Autodesk Fusion 360 part; units mm, degrees
(part 14 of 25)
  arc A3423 (31.4192, 17.8599) -> (31.5407, 18.1532) centre (31.4799, 18.0065) ccw
  line L1201 (39.8479, 17.8026) -> (39.6555, 17.6628)
  arc A3424 (36.7177, 17.8488) -> (36.9423, 17.6243) centre (36.83, 17.7366) ccw
  arc A3425 (41.043, 18.1351) -> (40.9448, 17.8331) centre (40.9939, 17.9841) ccw
  line L1202 (37.7489, 18.2753) -> (37.1, 18.0065)
  line L1203 (38.4511, 18.2753) -> (37.7489, 18.2753)
  arc A3426 (39.7677, 17.5505) -> (39.5432, 17.775) centre (39.6555, 17.6627) ccw
  arc A3427 (40.64, 18.18) -> (40.64, 17.8625) centre (40.64, 18.0212) ccw
  arc A3428 (40.7988, 18.0213) -> (40.4813, 18.0213) centre (40.6401, 18.0213) ccw
  arc A3429 (38.5119, 18.422) -> (38.3904, 18.1286) centre (38.4511, 18.2753) ccw
  arc A3430 (40.64, 16.3513) -> (40.64, 16.6688) centre (40.64, 16.51) ccw
  arc A3431 (40.5459, 17.8645) -> (40.4962, 18.1781) centre (40.5211, 18.0213) ccw
  arc A3432 (40.2613, 18.1409) -> (40.3109, 17.8273) centre (40.2861, 17.9841) ccw
  line L1204 (40.9939, 17.9841) -> (40.7589, 18.0213)
  arc A3433 (41.9212, 17.5879) -> (41.6643, 17.4012) centre (41.7927, 17.4945) ccw
  arc A3434 (40.9691, 17.8273) -> (41.0187, 18.1409) centre (40.9939, 17.9841) ccw
  line L1205 (35.9111, 18.2753) -> (35.2089, 18.2753)
  arc A3435 (27.5889, 18.434) -> (27.5889, 18.1165) centre (27.5889, 18.2752) ccw
  arc A3436 (26.5577, 17.6243) -> (26.7823, 17.8488) centre (26.67, 17.7366) ccw
  arc A3437 (29.0522, 18.1188) -> (28.8277, 17.8943) centre (28.94, 18.0065) ccw
  arc A3438 (30.8311, 18.1165) -> (30.8311, 18.434) centre (30.8311, 18.2752) ccw
  arc A3439 (36.7177, 17.6243) -> (36.9423, 17.8488) centre (36.83, 17.7366) ccw
  arc A3440 (36.6722, 18.1188) -> (36.4477, 17.8943) centre (36.56, 18.0066) ccw
  arc A3441 (29.0977, 17.8488) -> (29.3223, 17.6243) centre (29.21, 17.7366) ccw
  arc A3442 (28.3519, 18.422) -> (28.2304, 18.1286) centre (28.2911, 18.2753) ccw
  arc A3443 (33.9592, 17.8599) -> (34.0807, 18.1532) centre (34.02, 18.0065) ccw
  arc A3444 (33.4319, 18.422) -> (33.3104, 18.1286) centre (33.3712, 18.2753) ccw
  line L1206 (31.48, 18.0065) -> (30.8311, 18.2753)
  line L1207 (26.67, 17.7365) -> (26.4, 18.0065)
  line L1208 (28.94, 18.0065) -> (28.2911, 18.2753)
  line L1209 (32.6689, 18.2753) -> (32.02, 18.0065)
  arc A3445 (32.1323, 17.8943) -> (31.9078, 18.1188) centre (32.0201, 18.0066) ccw
  line L1210 (28.2911, 18.2753) -> (27.5889, 18.2753)
  arc A3446 (31.9593, 18.1532) -> (32.0808, 17.8599) centre (32.0201, 18.0066) ccw
  arc A3447 (34.1322, 18.1188) -> (33.9077, 17.8943) centre (34.02, 18.0066) ccw
  arc A3448 (35.2089, 18.434) -> (35.2089, 18.1165) centre (35.2089, 18.2752) ccw
  arc A3449 (26.8793, 18.1532) -> (27.0008, 17.8599) centre (26.9401, 18.0065) ccw
  line L1211 (34.29, 17.7365) -> (34.02, 18.0065)
  arc A3450 (32.7296, 18.1286) -> (32.6081, 18.422) centre (32.6688, 18.2753) ccw
  arc A3451 (30.1896, 18.1286) -> (30.0681, 18.422) centre (30.1288, 18.2753) ccw
  arc A3452 (30.8919, 18.422) -> (30.7704, 18.1286) centre (30.8312, 18.2753) ccw
  line L1212 (34.56, 18.0065) -> (34.29, 17.7365)
  arc A3453 (29.5923, 17.8943) -> (29.3678, 18.1188) centre (29.4801, 18.0066) ccw
  line L1213 (30.1289, 18.2753) -> (29.48, 18.0065)
  line L1214 (29.48, 18.0065) -> (29.21, 17.7365)
  line L1215 (36.83, 17.7365) -> (36.56, 18.0065)
  arc A3454 (35.9111, 18.1165) -> (35.9111, 18.434) centre (35.9111, 18.2752) ccw
  arc A3455 (35.9719, 18.422) -> (35.8504, 18.1286) centre (35.9112, 18.2753) ccw
  arc A3456 (33.3711, 18.1165) -> (33.3711, 18.434) centre (33.3711, 18.2752) ccw
  line L1216 (35.2089, 18.2753) -> (34.56, 18.0065)
  arc A3457 (26.5122, 18.1188) -> (26.2877, 17.8943) centre (26.4, 18.0066) ccw
  arc A3458 (34.1777, 17.6243) -> (34.4023, 17.8488) centre (34.29, 17.7366) ccw
  line L1217 (34.02, 18.0065) -> (33.3711, 18.2753)
  arc A3459 (16.3815, 13.6963) -> (16.26, 13.9897) centre (16.3208, 13.843) ccw
  arc A3460 (31.6377, 17.8488) -> (31.8623, 17.6243) centre (31.75, 17.7366) ccw
  line L1218 (15.9006, 13.669) -> (15.5791, 13.3475)
  line L1219 (27.5889, 18.2753) -> (26.94, 18.0065)
  arc A3461 (15.4669, 13.4597) -> (15.6914, 13.2352) centre (15.5792, 13.3475) ccw
  arc A3462 (28.2911, 18.1165) -> (28.2911, 18.434) centre (28.2911, 18.2752) ccw
  line L1220 (21.3635, 15.51) -> (21.717, 15.1565)
  line L1221 (36.56, 18.0065) -> (35.9111, 18.2753)
  arc A3463 (28.8792, 17.8599) -> (29.0007, 18.1532) centre (28.94, 18.0065) ccw
  line L1222 (32.02, 18.0065) -> (31.75, 17.7365)
  line L1223 (26.4, 18.0065) -> (25.7511, 18.2753)
  arc A3464 (31.6377, 17.6243) -> (31.8623, 17.8488) centre (31.75, 17.7366) ccw
  arc A3465 (29.4193, 18.1532) -> (29.5408, 17.8599) centre (29.4801, 18.0065) ccw
  line L1224 (30.8311, 18.2753) -> (30.1289, 18.2753)
  arc A3466 (36.4992, 17.8599) -> (36.6207, 18.1532) centre (36.56, 18.0065) ccw
  arc A3467 (35.2696, 18.1286) -> (35.1481, 18.422) centre (35.2088, 18.2753) ccw
  arc A3468 (27.0523, 17.8943) -> (26.8278, 18.1188) centre (26.9401, 18.0066) ccw
  arc A3469 (29.0977, 17.6243) -> (29.3223, 17.8488) centre (29.21, 17.7366) ccw
  arc A3470 (30.1289, 18.434) -> (30.1289, 18.1165) centre (30.1289, 18.2752) ccw
  arc A3471 (31.5922, 18.1188) -> (31.3677, 17.8943) centre (31.4799, 18.0066) ccw
  line L1225 (33.3711, 18.2753) -> (32.6689, 18.2753)
  arc A3472 (34.4993, 18.1532) -> (34.6208, 17.8599) centre (34.5601, 18.0065) ccw
  arc A3473 (25.7511, 18.1165) -> (25.7511, 18.434) centre (25.7511, 18.2752) ccw
  arc A3474 (23.9722, 18.1188) -> (23.7477, 17.8943) centre (23.86, 18.0065) ccw
  line L1226 (25.0489, 18.2753) -> (24.4, 18.0065)
  arc A3475 (16.0129, 13.5567) -> (15.7884, 13.7812) centre (15.9007, 13.6689) ccw
  line L1227 (21.0947, 16.8611) -> (21.0947, 16.1589)
  arc A3476 (21.9723, 17.8943) -> (21.7478, 18.1188) centre (21.8601, 18.0066) ccw
  arc A3477 (21.7993, 18.1532) -> (21.9208, 17.8599) centre (21.8601, 18.0065) ccw
  arc A3478 (23.2111, 18.1165) -> (23.2111, 18.434) centre (23.2111, 18.2752) ccw
  line L1228 (14.6499, 12.9032) -> (13.7795, 12.0328)
  arc A3479 (25.8119, 18.422) -> (25.6904, 18.1286) centre (25.7512, 18.2753) ccw
  line L1229 (21.0947, 16.1589) -> (21.3635, 15.51)
  arc A3480 (21.2535, 16.8611) -> (20.9359, 16.8611) centre (21.0947, 16.8611) ccw
  arc A3481 (15.6914, 13.2352) -> (15.4669, 13.4597) centre (15.5792, 13.3475) ccw
  arc A3482 (21.5101, 17.4492) -> (21.2168, 17.5707) centre (21.3635, 17.5099) ccw
  arc A3483 (24.3393, 18.1532) -> (24.4608, 17.8599) centre (24.4001, 18.0065) ccw
  arc A3484 (21.2414, 16.2196) -> (20.948, 16.0981) centre (21.0947, 16.1589) ccw
  line L1230 (23.86, 18.0065) -> (23.2111, 18.2753)
  line L1231 (21.1166, 13.843) -> (16.3207, 13.843)
  arc A3485 (22.5696, 18.1286) -> (22.4481, 18.422) centre (22.5089, 18.2753) ccw
  line L1232 (21.86, 18.0065) -> (21.3635, 17.51)
  arc A3486 (21.8758, 15.1565) -> (21.5583, 15.1565) centre (21.717, 15.1565) ccw
  line L1233 (21.717, 14.4434) -> (21.1166, 13.843)
  arc A3487 (23.2719, 18.422) -> (23.1504, 18.1286) centre (23.2111, 18.2753) ccw
  arc A3488 (22.5089, 18.434) -> (22.5089, 18.1165) centre (22.5089, 18.2752) ccw
  line L1234 (15.5791, 13.3475) -> (15.1349, 12.9032)
  arc A3489 (13.6672, 12.145) -> (13.8918, 11.9205) centre (13.7795, 12.0328) ccw
  arc A3490 (20.948, 16.9219) -> (21.2414, 16.8004) centre (21.0947, 16.8612) ccw
  arc A3491 (13.6208, 10.8018) -> (13.9383, 10.8018) centre (13.7796, 10.8018) ccw
  line L1235 (24.13, 17.7365) -> (23.86, 18.0065)
  line L1236 (21.3635, 17.51) -> (21.0947, 16.8611)
  arc A3492 (21.0043, 13.9553) -> (21.2288, 13.7307) centre (21.1165, 13.843) ccw
  arc A3493 (21.5583, 14.4434) -> (21.8758, 14.4434) centre (21.717, 14.4434) ccw
  arc A3494 (21.8293, 14.3312) -> (21.6047, 14.5557) centre (21.717, 14.4435) ccw
  arc A3495 (21.2168, 15.4493) -> (21.5101, 15.5708) centre (21.3635, 15.51) ccw
  arc A3496 (23.7992, 17.8599) -> (23.9207, 18.1532) centre (23.8599, 18.0065) ccw
  line L1237 (22.5089, 18.2753) -> (21.86, 18.0065)
  arc A3497 (25.0489, 18.434) -> (25.0489, 18.1165) centre (25.0489, 18.2752) ccw
  arc A3498 (24.0177, 17.8488) -> (24.2423, 17.6243) centre (24.13, 17.7366) ccw
  arc A3499 (15.1349, 12.7444) -> (15.1349, 13.0619) centre (15.1349, 12.9032) ccw
  arc A3500 (21.4757, 15.6223) -> (21.2512, 15.3978) centre (21.3635, 15.51) ccw
  arc A3501 (15.8399, 13.8157) -> (15.9614, 13.5223) centre (15.9007, 13.669) ccw
  arc A3502 (14.6499, 13.0619) -> (14.6499, 12.7444) centre (14.6499, 12.9032) ccw
  arc A3503 (24.0177, 17.6243) -> (24.2423, 17.8488) centre (24.13, 17.7366) ccw
  line L1238 (24.4, 18.0065) -> (24.13, 17.7365)
  arc A3504 (20.9359, 16.1589) -> (21.2535, 16.1589) centre (21.0947, 16.1589) ccw
  arc A3505 (26.3392, 17.8599) -> (26.4607, 18.1532) centre (26.3999, 18.0065) ccw
  arc A3506 (15.0226, 13.0155) -> (15.2471, 12.7909) centre (15.1349, 12.9032) ccw
  line L1239 (21.717, 15.1565) -> (21.717, 14.4434)
  line L1240 (25.7511, 18.2753) -> (25.0489, 18.2753)
  arc A3507 (14.7622, 12.7909) -> (14.5377, 13.0155) centre (14.65, 12.9032) ccw
  arc A3508 (25.1096, 18.1286) -> (24.9881, 18.422) centre (25.0489, 18.2753) ccw
  arc A3509 (21.2512, 17.6222) -> (21.4757, 17.3977) centre (21.3635, 17.5099) ccw
  line L1241 (13.7795, 12.0328) -> (13.7795, 10.8018)
  line L1242 (23.2111, 18.2753) -> (22.5089, 18.2753)
  line L1243 (15.1349, 12.9032) -> (14.6499, 12.9032)
  arc A3510 (24.5123, 17.8943) -> (24.2878, 18.1188) centre (24.4001, 18.0066) ccw
  arc A3511 (65.9384, 2.7686) -> (65.9384, 2.7178) centre (65.9384, 2.7432) ccw
  arc A3512 (66.0553, 2.2782) -> (66.0811, 2.2345) centre (66.0682, 2.2564) ccw
  arc A3513 (63.0301, 1.5494) -> (63.0301, 1.6002) centre (63.0301, 1.5748) ccw
  arc A3514 (57.5748, 1.5748) -> (57.6256, 1.5748) centre (57.6002, 1.5748) ccw
  arc A3515 (66.1981, 2.4836) -> (65.9384, 2.7432) centre (65.9384, 2.4835) ccw
  arc A3516 (65.556, 1.8344) -> (65.6068, 1.8344) centre (65.5814, 1.8344) ccw
  arc A3517 (58.2027, 1.5748) -> (58.2535, 1.5748) centre (58.2281, 1.5748) ccw
  line L1244 (55.3077, 1.5748) -> (55.827, 1.5748)
  arc A3518 (55.4375, 2.2493) -> (55.4375, 2.1985) centre (55.4375, 2.2239) ccw
  arc A3519 (65.1543, 2.4836) -> (65.1035, 2.4836) centre (65.1289, 2.4836) ccw
  arc A3520 (58.9026, 2.7432) -> (58.8518, 2.7432) centre (58.8772, 2.7432) ccw
  arc A3521 (55.8524, 2.7432) -> (55.8016, 2.7432) centre (55.827, 2.7432) ccw
  arc A3522 (63.0142, 2.4637) -> (63.046, 2.5034) centre (63.0301, 2.4835) ccw
  line L1245 (54.5067, 2.0941) -> (54.8313, 2.0941)
  arc A3523 (56.6617, 1.5668) -> (56.7099, 1.5828) centre (56.6858, 1.5748) ccw
  arc A3524 (61.238, 1.6002) -> (61.238, 1.5494) centre (61.238, 1.5748) ccw
  line L1246 (57.73, 1.5748) -> (57.4703, 1.5748)
  arc A3525 (55.827, 2.1985) -> (55.827, 2.2493) centre (55.827, 2.2239) ccw
  arc A3526 (54.1594, 1.5862) -> (54.2049, 1.5634) centre (54.1822, 1.5748) ccw
  arc A3527 (55.3077, 1.6002) -> (55.3077, 1.5494) centre (55.3077, 1.5748) ccw
  arc A3528 (54.8313, 2.0687) -> (54.8313, 2.1195) centre (54.8313, 2.0941) ccw
  line L1247 (55.827, 1.5748) -> (55.827, 2.7432)
  arc A3529 (63.524, 1.6002) -> (63.524, 1.5494) centre (63.524, 1.5748) ccw
  arc A3530 (66.2234, 2.4836) -> (66.1727, 2.4836) centre (66.1981, 2.4836) ccw
  arc A3531 (65.6311, 2.6662) -> (65.6615, 2.6255) centre (65.6463, 2.6459) ccw
  line L1248 (59.4473, 1.8994) -> (59.4473, 2.7432)
  arc A3532 (56.6617, 1.5828) -> (56.7099, 1.5668) centre (56.6858, 1.5748) ccw
  arc A3533 (53.11, 1.8344) -> (53.0592, 1.8344) centre (53.0846, 1.8344) ccw
  arc A3534 (53.0846, 1.8344) -> (53.3443, 1.5748) centre (53.3443, 1.8345) ccw
  arc A3535 (66.0804, 2.2341) -> (66.0561, 2.2787) centre (66.0682, 2.2564) ccw
  line L1249 (58.8772, 2.7432) -> (58.2281, 1.5748)
  arc A3536 (53.3443, 1.5494) -> (53.3443, 1.6002) centre (53.3443, 1.5748) ccw
  line L1250 (54.1822, 1.5748) -> (54.4418, 2.0941)
  arc A3537 (57.0993, 2.7352) -> (57.0511, 2.7512) centre (57.0752, 2.7432) ccw
  arc A3538 (53.3443, 1.5748) -> (53.7337, 1.7371) centre (53.3442, 2.1232) ccw
  line L1251 (57.0752, 2.7432) -> (56.6858, 1.5748)
  line L1252 (56.6858, 1.5748) -> (56.2963, 2.7432)
  arc A3539 (64.1731, 1.5494) -> (64.1731, 1.6002) centre (64.1731, 1.5748) ccw
  line L1253 (61.8871, 2.4836) -> (61.5626, 2.7432)
  arc A3540 (61.8871, 1.5494) -> (61.8871, 1.6002) centre (61.8871, 1.5748) ccw
  line L1254 (65.1289, 1.8344) -> (65.1289, 2.4836)
  arc A3541 (54.4645, 2.0827) -> (54.4191, 2.1054) centre (54.4418, 2.0941) ccw
  line L1255 (55.827, 2.2239) -> (55.4375, 2.2239)
  arc A3542 (53.3443, 1.6002) -> (53.3443, 1.5494) centre (53.3443, 1.5748) ccw
  arc A3543 (64.1572, 2.4637) -> (64.189, 2.5034) centre (64.1731, 2.4835) ccw
  line L1256 (64.1731, 1.5748) -> (63.524, 1.5748)
  arc A3544 (66.2485, 1.7192) -> (66.2125, 1.755) centre (66.2305, 1.7371) ccw
  arc A3545 (65.1543, 1.8344) -> (65.1035, 1.8344) centre (65.1289, 1.8344) ccw
  line L1257 (64.8693, 2.7432) -> (64.6096, 2.7432)
  arc A3546 (64.8693, 1.5748) -> (65.1289, 1.8344) centre (64.8693, 1.8344) ccw
  arc A3547 (63.8644, 2.763) -> (63.8327, 2.7234) centre (63.8485, 2.7432) ccw
  arc A3548 (65.1289, 2.4836) -> (64.8693, 2.7432) centre (64.8693, 2.4836) ccw
  arc A3549 (63.8232, 1.5748) -> (63.874, 1.5748) centre (63.8486, 1.5748) ccw
  arc A3550 (66.0682, 2.2564) -> (66.1981, 2.4836) centre (65.9344, 2.4836) ccw
  arc A3551 (62.381, 1.6002) -> (62.381, 1.5494) centre (62.381, 1.5748) ccw
  arc A3552 (61.5372, 1.5748) -> (61.588, 1.5748) centre (61.5626, 1.5748) ccw
  arc A3553 (61.5784, 2.763) -> (61.5467, 2.7234) centre (61.5625, 2.7432) ccw
  line L1258 (60.0964, 2.7432) -> (60.0964, 1.8994)
  arc A3554 (65.9384, 2.7432) -> (65.6463, 2.6458) centre (65.9384, 2.2564) ccw
  line L1259 (61.5626, 2.7432) -> (61.5626, 1.5748)
  arc A3555 (54.5067, 2.1195) -> (54.5067, 2.0687) centre (54.5067, 2.0941) ccw
  line L1260 (58.2281, 1.5748) -> (58.2281, 2.7432)
  arc A3556 (57.4703, 1.6002) -> (57.4703, 1.5494) centre (57.4703, 1.5748) ccw
  line L1261 (65.7112, 2.0616) -> (66.0682, 2.2564)
  arc A3557 (64.8693, 2.7178) -> (64.8693, 2.7686) centre (64.8693, 2.7432) ccw
  arc A3558 (64.6096, 1.6002) -> (64.6096, 1.5494) centre (64.6096, 1.5748) ccw
  arc A3559 (65.1035, 1.8344) -> (65.1543, 1.8344) centre (65.1289, 1.8344) ccw
  line L1262 (63.0301, 1.5748) -> (62.381, 1.5748)
  arc A3560 (61.588, 2.7432) -> (61.5372, 2.7432) centre (61.5626, 2.7432) ccw
  arc A3561 (60.071, 1.8994) -> (60.1218, 1.8994) centre (60.0964, 1.8994) ccw
  arc A3562 (62.7214, 2.763) -> (62.6897, 2.7234) centre (62.7055, 2.7432) ccw
  arc A3563 (65.9384, 2.7178) -> (65.9384, 2.7686) centre (65.9384, 2.7432) ccw
  line L1263 (64.6096, 1.5748) -> (64.8693, 1.5748)
  arc A3564 (65.5814, 1.8344) -> (65.841, 1.5748) centre (65.841, 1.8344) ccw
  arc A3565 (66.1727, 2.4836) -> (66.2235, 2.4836) centre (66.1981, 2.4836) ccw
  arc A3566 (60.1218, 2.7432) -> (60.071, 2.7432) centre (60.0964, 2.7432) ccw
  arc A3567 (65.6068, 1.8344) -> (65.556, 1.8344) centre (65.5814, 1.8344) ccw
  arc A3568 (64.8693, 1.6002) -> (64.8693, 1.5494) centre (64.8693, 1.5748) ccw
  arc A3569 (65.7112, 2.0616) -> (65.5814, 1.8344) centre (65.8451, 1.8344) ccw
  arc A3570 (66.96, 2.7432) -> (66.9092, 2.7432) centre (66.9346, 2.7432) ccw
  arc A3571 (66.6101, 2.7686) -> (66.6101, 2.7178) centre (66.6101, 2.7432) ccw
  line L1264 (67.2592, 2.7432) -> (66.6101, 2.7432)
  arc A3572 (65.841, 1.5494) -> (65.841, 1.6002) centre (65.841, 1.5748) ccw
  arc A3573 (62.6802, 1.5748) -> (62.731, 1.5748) centre (62.7056, 1.5748) ccw
  line L1265 (63.0301, 2.4836) -> (62.7056, 2.7432)
  arc A3574 (61.8712, 2.4637) -> (61.903, 2.5034) centre (61.8871, 2.4835) ccw
  arc A3575 (67.2592, 2.7178) -> (67.2592, 2.7686) centre (67.2592, 2.7432) ccw
  arc A3576 (65.1035, 2.4836) -> (65.1543, 2.4836) centre (65.1289, 2.4836) ccw
  arc A3577 (64.8693, 1.5494) -> (64.8693, 1.6002) centre (64.8693, 1.5748) ccw
  line L1266 (62.7056, 2.7432) -> (62.7056, 1.5748)
  arc A3578 (65.841, 1.6002) -> (65.841, 1.5494) centre (65.841, 1.5748) ccw
  arc A3579 (66.9092, 1.5748) -> (66.96, 1.5748) centre (66.9346, 1.5748) ccw
  arc A3580 (59.4473, 1.8994) -> (60.0964, 1.8994) centre (59.7719, 1.8994) ccw
  line L1267 (64.1731, 2.4836) -> (63.8486, 2.7432)
  arc A3581 (65.7241, 2.0397) -> (65.6983, 2.0835) centre (65.7112, 2.0616) ccw
  line L1268 (61.8871, 1.5748) -> (61.238, 1.5748)
  arc A3582 (65.6991, 2.0839) -> (65.7234, 2.0393) centre (65.7113, 2.0616) ccw
  line L1269 (63.8486, 2.7432) -> (63.8486, 1.5748)
  arc A3583 (62.731, 2.7432) -> (62.6802, 2.7432) centre (62.7056, 2.7432) ccw
  arc A3584 (65.841, 1.5748) -> (66.2305, 1.7371) centre (65.841, 2.1233) ccw
  arc A3585 (60.1218, 1.8994) -> (60.071, 1.8994) centre (60.0964, 1.8994) ccw
  arc A3586 (64.6096, 2.7686) -> (64.6096, 2.7178) centre (64.6096, 2.7432) ccw
  line L1270 (66.9346, 1.5748) -> (66.9346, 2.7432)
  arc A3587 (64.8693, 2.7686) -> (64.8693, 2.7178) centre (64.8693, 2.7432) ccw
  arc A3588 (63.874, 2.7432) -> (63.8232, 2.7432) centre (63.8486, 2.7432) ccw
  arc A3589 (59.4727, 1.8994) -> (59.4219, 1.8994) centre (59.4473, 1.8994) ccw
  arc A3590 (39.4305, 29.7091) -> (39.7238, 29.8306) centre (39.5772, 29.7698) ccw
  line L1271 (38.7475, 29.511) -> (39.41, 30.1735)
  line L1272 (52.2496, 23.4133) -> (52.3555, 23.3074)
  line L1273 (53.2211, 22.9489) -> (53.34, 22.9489)
  arc A3591 (53.1962, 22.7921) -> (53.2459, 23.1057) centre (53.2211, 22.9489) ccw
  arc A3592 (52.6878, 22.9182) -> (52.8319, 23.2011) centre (52.7599, 23.0597) ccw
  arc A3593 (47.9089, 22.8537) -> (47.9089, 22.5361) centre (47.9089, 22.6949) ccw
  line L1274 (28.1196, 27.3867) -> (27.813, 27.6933)
  arc A3594 (53.34, 22.7902) -> (53.34, 23.1077) centre (53.34, 22.9489) ccw
  arc A3595 (47.1478, 22.8514) -> (47.3723, 23.0759) centre (47.2601, 22.9636) ccw
  line L1275 (45.5255, 24.4221) -> (46.4947, 24.4221)
  line L1276 (52.9861, 22.9861) -> (53.2211, 22.9489)
  arc A3596 (52.4488, 23.4359) -> (52.2621, 23.179) centre (52.3555, 23.3075) ccw
  arc A3597 (52.2432, 23.1952) -> (52.4677, 23.4197) centre (52.3555, 23.3075) ccw
  arc A3598 (53.0109, 23.1429) -> (52.9613, 22.8293) centre (52.9861, 22.9861) ccw
  arc A3599 (47.3208, 23.1103) -> (47.1993, 22.817) centre (47.2601, 22.9636) ccw
  arc A3600 (47.8481, 22.5482) -> (47.9696, 22.8416) centre (47.9089, 22.6949) ccw
  arc A3601 (39.6894, 29.8821) -> (39.4649, 29.6576) centre (39.5772, 29.7699) ccw
  arc A3602 (52.62, 23.3091) -> (52.4758, 23.0262) centre (52.5479, 23.1677) ccw
  arc A3603 (29.3289, 27.6923) -> (29.3289, 28.0098) centre (29.3289, 27.8511) ccw
  arc A3604 (27.9717, 28.7366) -> (27.6542, 28.7366) centre (27.813, 28.7366) ccw
  arc A3605 (40.3906, 29.3851) -> (40.3906, 29.0676) centre (40.3906, 29.2264) ccw
  line L1277 (49.26, 22.9637) -> (49.53, 23.2337)
  line L1278 (46.4947, 24.4221) -> (46.4947, 24.1091)
  arc A3606 (52.3619, 23.301) -> (52.1373, 23.5255) centre (52.2496, 23.4133) ccw
  arc A3607 (52.8089, 23.2106) -> (52.7108, 22.9086) centre (52.7599, 23.0596) ccw
  arc A3608 (49.8608, 23.1103) -> (49.7393, 22.817) centre (49.8, 22.9637) ccw
  arc A3609 (29.0911, 28.0098) -> (29.0911, 27.6923) centre (29.0911, 27.8511) ccw
  line L1279 (39.9298, 29.4172) -> (40.3906, 29.2263)
  arc A3610 (39.5566, 30.2343) -> (39.2633, 30.1128) centre (39.41, 30.1736) ccw
  line L1280 (29.3289, 27.8511) -> (29.21, 27.8511)
  arc A3611 (50.4489, 22.8537) -> (50.4489, 22.5361) centre (50.4489, 22.6949) ccw
  arc A3612 (52.937, 22.8351) -> (53.0352, 23.1371) centre (52.9861, 22.9861) ccw
  arc A3613 (38.2666, 29.4837) -> (38.3881, 29.1903) centre (38.3274, 29.337) ccw
  line L1281 (46.7634, 23.4602) -> (47.26, 22.9637)
  line L1282 (51.8, 22.9637) -> (52.2496, 23.4133)
  line L1283 (52.7599, 23.0596) -> (52.9861, 22.9861)
  arc A3614 (51.0904, 22.8416) -> (51.2119, 22.5482) centre (51.1512, 22.6949) ccw
  line L1284 (52.5479, 23.1676) -> (52.7599, 23.0596)
  line L1285 (52.3555, 23.3074) -> (52.5479, 23.1676)
  arc A3615 (52.4546, 23.0392) -> (52.6412, 23.296) centre (52.5479, 23.1676) ccw
  line L1286 (40.5107, 29.2263) -> (45.1661, 24.571)
  line L1287 (49.8, 22.9637) -> (50.4489, 22.6949)
  arc A3616 (45.4647, 24.2754) -> (45.5862, 24.5688) centre (45.5255, 24.4221) ccw
  arc A3617 (46.6414, 24.1698) -> (46.348, 24.0483) centre (46.4947, 24.1091) ccw
  line L1288 (40.3906, 29.2263) -> (40.5107, 29.2263)
  arc A3618 (29.3538, 28.0079) -> (29.3041, 27.6943) centre (29.329, 27.8511) ccw
  line L1289 (53.34, 22.9489) -> (53.34, 25.4)
  arc A3619 (52.3619, 23.5255) -> (52.1373, 23.301) centre (52.2496, 23.4132) ccw
  arc A3620 (51.6877, 23.0759) -> (51.9122, 22.8514) centre (51.7999, 22.9637) ccw
  arc A3621 (49.1477, 23.0759) -> (49.3722, 22.8514) centre (49.26, 22.9637) ccw
  arc A3622 (40.5107, 29.0676) -> (40.5107, 29.3851) centre (40.5107, 29.2264) ccw
  arc A3623 (46.8757, 23.5725) -> (46.6512, 23.348) centre (46.7635, 23.4603) ccw
  arc A3624 (53.2211, 23.1077) -> (53.2211, 22.7902) centre (53.2211, 22.9489) ccw
  line L1290 (47.26, 22.9637) -> (47.9089, 22.6949)
  arc A3625 (45.2268, 24.7176) -> (45.1053, 24.4243) centre (45.166, 24.5709) ccw
  arc A3626 (51.8607, 22.817) -> (51.7392, 23.1103) centre (51.7999, 22.9637) ccw
  arc A3627 (48.6111, 22.5361) -> (48.6111, 22.8537) centre (48.6111, 22.6949) ccw
  arc A3628 (46.4947, 24.2633) -> (46.4947, 24.5809) centre (46.4947, 24.4221) ccw
  arc A3629 (45.5255, 24.5809) -> (45.5255, 24.2633) centre (45.5255, 24.4221) ccw
  arc A3630 (49.3207, 22.817) -> (49.1992, 23.1103) centre (49.26, 22.9637) ccw
  line L1291 (46.4947, 24.1091) -> (46.7634, 23.4602)
  arc A3631 (48.5504, 22.8416) -> (48.6719, 22.5482) centre (48.6112, 22.6949) ccw
  arc A3632 (45.0538, 24.4587) -> (45.2783, 24.6832) centre (45.166, 24.571) ccw
  line L1292 (48.6111, 22.6949) -> (49.26, 22.9637)
  arc A3633 (53.4988, 25.4) -> (53.1813, 25.4) centre (53.3401, 25.4) ccw
  line L1293 (49.53, 23.2337) -> (49.8, 22.9637)
  arc A3634 (53.1813, 22.9489) -> (53.4988, 22.9489) centre (53.3401, 22.9489) ccw
  line L1294 (54.7406, 23.8801) -> (54.8141, 24.1063)
  arc A3635 (53.4987, 25.4) -> (53.1812, 25.4) centre (53.34, 25.4) ccw
  arc A3636 (54.761, 23.5748) -> (54.5041, 23.7614) centre (54.6326, 23.6681) ccw
  arc A3637 (54.8513, 25.2413) -> (54.8513, 25.5588) centre (54.8513, 25.4001) ccw
  line L1295 (50.4489, 22.6949) -> (51.1511, 22.6949)
  arc A3638 (51.1511, 22.5361) -> (51.1511, 22.8537) centre (51.1511, 22.6949) ccw
  line L1296 (51.1511, 22.6949) -> (51.8, 22.9637)
  arc A3639 (46.336, 24.1091) -> (46.6534, 24.1091) centre (46.4947, 24.1091) ccw
  line L1297 (54.6326, 23.6681) -> (54.7406, 23.8801)
  line L1298 (54.1321, 23.1676) -> (54.3245, 23.3074)
  arc A3640 (53.34, 23.1077) -> (53.34, 22.7902) centre (53.34, 22.9489) ccw
  arc A3641 (46.6168, 23.3995) -> (46.9101, 23.521) centre (46.7634, 23.4603) ccw
  arc A3642 (54.6631, 26.6446) -> (54.9651, 26.7428) centre (54.8141, 26.6937) ccw
  line L1299 (54.4928, 23.4757) -> (54.6326, 23.6681)
  line L1300 (53.4589, 22.9489) -> (53.6939, 22.9861)
  arc A3643 (54.882, 23.808) -> (54.5991, 23.9521) centre (54.7405, 23.8801) ccw
  line L1301 (47.9089, 22.6949) -> (48.6111, 22.6949)
  arc A3644 (50.3881, 22.5482) -> (50.5096, 22.8416) centre (50.4489, 22.6949) ccw
  arc A3645 (54.2042, 23.0262) -> (54.06, 23.3091) centre (54.1321, 23.1677) ccw
  arc A3646 (49.6878, 22.8514) -> (49.9123, 23.0759) centre (49.8, 22.9637) ccw
  arc A3647 (55.0081, 24.3164) -> (54.6945, 24.3661) centre (54.8513, 24.3413) ccw
  arc A3648 (54.8513, 25.2412) -> (54.8513, 25.5587) centre (54.8513, 25.4) ccw
  line L1302 (53.34, 25.4) -> (54.8513, 25.4)
  arc A3649 (54.6945, 26.4339) -> (55.0081, 26.4836) centre (54.8513, 26.4588) ccw
  arc A3650 (46.6534, 24.4221) -> (46.336, 24.4221) centre (46.4947, 24.4221) ccw
  arc A3651 (49.6423, 23.1214) -> (49.4177, 23.3459) centre (49.53, 23.2336) ccw
  line L1303 (54.8141, 26.6937) -> (54.7406, 26.9199)
  arc A3652 (53.4341, 23.1057) -> (53.4838, 22.7921) centre (53.459, 22.9489) ccw
  arc A3653 (54.6925, 24.3413) -> (55.01, 24.3413) centre (54.8513, 24.3413) ccw
  line L1304 (54.8513, 25.4) -> (54.8513, 26.4587)
  arc A3654 (53.7187, 22.8293) -> (53.6691, 23.1429) centre (53.6939, 22.9861) ccw
  line L1305 (54.8513, 26.4587) -> (54.8141, 26.6937)
  arc A3655 (53.4589, 22.7902) -> (53.4589, 23.1077) centre (53.4589, 22.9489) ccw
  arc A3656 (54.5041, 27.0386) -> (54.761, 27.2252) centre (54.6326, 27.1319) ccw
  line L1306 (53.34, 25.4) -> (53.34, 22.9489)
  arc A3657 (54.9651, 24.0572) -> (54.6631, 24.1554) centre (54.8141, 24.1063) ccw
  arc A3658 (53.1813, 25.4) -> (53.4988, 25.4) centre (53.3401, 25.4) ccw
  arc A3659 (55.01, 26.4587) -> (54.6925, 26.4587) centre (54.8513, 26.4587) ccw
  arc A3660 (53.9692, 22.9086) -> (53.8711, 23.2106) centre (53.9201, 23.0596) ccw
  arc A3661 (49.6423, 23.3459) -> (49.4177, 23.1214) centre (49.53, 23.2336) ccw
  line L1307 (54.8513, 25.4) -> (53.34, 25.4)
  line L1308 (54.8141, 24.1063) -> (54.8513, 24.3413)
  line L1309 (54.4928, 27.3243) -> (54.3245, 27.4926)
  arc A3662 (53.34, 25.2412) -> (53.34, 25.5587) centre (53.34, 25.4) ccw
  line L1310 (54.7406, 26.9199) -> (54.6326, 27.1319)
  arc A3663 (54.9709, 26.7185) -> (54.6573, 26.6689) centre (54.8141, 26.6937) ccw
  arc A3664 (53.34, 25.5588) -> (53.34, 25.2413) centre (53.34, 25.4001) ccw
  line L1311 (54.8513, 24.3413) -> (54.8513, 25.4)
  line L1312 (45.1661, 24.571) -> (45.5255, 24.4221)
  arc A3665 (55.01, 25.4) -> (54.6925, 25.4) centre (54.8513, 25.4) ccw
  arc A3666 (40.623, 29.3386) -> (40.3985, 29.114) centre (40.5108, 29.2263) ccw
  arc A3667 (53.6448, 23.1371) -> (53.743, 22.8351) centre (53.6939, 22.9861) ccw
  arc A3668 (54.6212, 27.4177) -> (54.3643, 27.231) centre (54.4928, 27.3244) ccw
  arc A3669 (54.4179, 23.179) -> (54.2312, 23.4359) centre (54.3246, 23.3075) ccw
  arc A3670 (54.605, 23.3634) -> (54.3805, 23.5879) centre (54.4928, 23.4757) ccw
  arc A3671 (54.3643, 23.569) -> (54.6212, 23.3823) centre (54.4928, 23.4757) ccw
  arc A3672 (54.5896, 23.9291) -> (54.8916, 23.831) centre (54.7406, 23.8801) ccw
  arc A3673 (53.8481, 23.2011) -> (53.9922, 22.9182) centre (53.9202, 23.0597) ccw
  arc A3674 (52.9613, 27.9707) -> (53.0109, 27.6571) centre (52.9861, 27.8139) ccw
  arc A3675 (53.1812, 25.4) -> (53.4987, 25.4) centre (53.34, 25.4) ccw
  arc A3676 (54.6573, 24.1311) -> (54.9709, 24.0815) centre (54.8141, 24.1063) ccw
  arc A3677 (54.774, 27.204) -> (54.4911, 27.0598) centre (54.6326, 27.1319) ccw
  arc A3678 (54.5991, 26.8479) -> (54.882, 26.992) centre (54.7405, 26.92) ccw
  arc A3679 (53.34, 25.5587) -> (53.34, 25.2412) centre (53.34, 25.4) ccw
  arc A3680 (54.0388, 23.296) -> (54.2254, 23.0392) centre (54.1321, 23.1676) ccw
  line L1313 (53.34, 22.9489) -> (53.4589, 22.9489)
  arc A3681 (54.4911, 23.7402) -> (54.774, 23.596) centre (54.6326, 23.6681) ccw
  arc A3682 (54.8916, 26.969) -> (54.5896, 26.8709) centre (54.7406, 26.92) ccw
  arc A3683 (47.2781, 34.3097) -> (47.1566, 34.0163) centre (47.2174, 34.163) ccw
  arc A3684 (47.5767, 33.8423) -> (47.6982, 34.1357) centre (47.6375, 33.989) ccw
  arc A3685 (53.743, 27.9649) -> (53.6448, 27.6629) centre (53.6939, 27.8139) ccw
  arc A3686 (47.8467, 33.5552) -> (48.0712, 33.7797) centre (47.959, 33.6675) ccw
  arc A3687 (54.06, 27.4909) -> (54.2042, 27.7738) centre (54.1321, 27.6324) ccw
  line L1314 (52.9861, 27.8139) -> (52.7599, 27.7404)
  arc A3688 (53.34, 25.5587) -> (53.34, 25.2412) centre (53.34, 25.4) ccw
  arc A3689 (53.6691, 27.6571) -> (53.7187, 27.9707) centre (53.6939, 27.8139) ccw
  arc A3690 (53.0352, 27.6629) -> (52.937, 27.9649) centre (52.9861, 27.8139) ccw
  line L1315 (54.3245, 23.3074) -> (54.4928, 23.4757)
  arc A3691 (53.4988, 27.8511) -> (53.1813, 27.8511) centre (53.3401, 27.8511) ccw
  arc A3692 (51.6567, 29.7452) -> (51.8812, 29.9697) centre (51.769, 29.8575) ccw
  line L1316 (54.3245, 27.4926) -> (54.1321, 27.6324)
  arc A3693 (52.1017, 29.4374) -> (51.7842, 29.4374) centre (51.943, 29.4374) ccw
  line L1317 (53.34, 25.4) -> (53.34, 27.8511)
  arc A3694 (52.4677, 27.3803) -> (52.2432, 27.6048) centre (52.3555, 27.4926) ccw
  arc A3695 (53.4589, 27.6923) -> (53.4589, 28.0098) centre (53.4589, 27.8511) ccw
  arc A3696 (53.2459, 27.6943) -> (53.1962, 28.0079) centre (53.221, 27.8511) ccw
  arc A3697 (53.1812, 22.9489) -> (53.4987, 22.9489) centre (53.34, 22.9489) ccw
  arc A3698 (53.4987, 27.8511) -> (53.1812, 27.8511) centre (53.34, 27.8511) ccw
  line L1318 (53.9201, 27.7404) -> (53.6939, 27.8139)
  arc A3699 (51.7963, 29.3766) -> (52.0897, 29.4981) centre (51.943, 29.4374) ccw
  arc A3700 (53.2211, 28.0098) -> (53.2211, 27.6923) centre (53.2211, 27.8511) ccw
  arc A3701 (52.4758, 27.7738) -> (52.62, 27.4909) centre (52.5479, 27.6323) ccw
  arc A3702 (54.2123, 23.4197) -> (54.4368, 23.1952) centre (54.3246, 23.3075) ccw
  arc A3703 (54.6925, 25.4) -> (55.01, 25.4) centre (54.8513, 25.4) ccw
  arc A3704 (51.7842, 27.6933) -> (52.1017, 27.6933) centre (51.943, 27.6933) ccw
  line L1319 (53.9201, 23.0596) -> (54.1321, 23.1676)
  arc A3705 (53.1813, 25.4) -> (53.4988, 25.4) centre (53.3401, 25.4) ccw
  arc A3706 (53.8711, 27.5894) -> (53.9692, 27.8914) centre (53.9202, 27.7404) ccw
  arc A3707 (53.34, 25.5588) -> (53.34, 25.2413) centre (53.34, 25.4001) ccw
  arc A3708 (54.2312, 27.3641) -> (54.4179, 27.621) centre (54.3246, 27.4925) ccw
  arc A3709 (52.6412, 27.5039) -> (52.4546, 27.7608) centre (52.5479, 27.6324) ccw
  line L1320 (53.2211, 27.8511) -> (52.9861, 27.8139)
  arc A3710 (52.8319, 27.5989) -> (52.6878, 27.8818) centre (52.7599, 27.7404) ccw
  line L1321 (52.5479, 27.6324) -> (52.3555, 27.4926)
  arc A3711 (53.9922, 27.8818) -> (53.8481, 27.5989) centre (53.9202, 27.7403) ccw
  line L1322 (54.6326, 27.1319) -> (54.4928, 27.3243)
  arc A3712 (53.34, 28.0098) -> (53.34, 27.6923) centre (53.34, 27.8511) ccw
  line L1323 (53.34, 27.8511) -> (53.34, 25.4)
  line L1324 (53.6939, 22.9861) -> (53.9201, 23.0596)
  arc A3713 (54.4368, 27.6048) -> (54.2123, 27.3803) centre (54.3246, 27.4925) ccw
  line L1325 (53.6939, 27.8139) -> (53.4589, 27.8511)
  arc A3714 (53.4988, 25.4) -> (53.1813, 25.4) centre (53.3401, 25.4) ccw
  arc A3715 (22.9777, 29.0302) -> (23.2022, 28.8056) centre (23.09, 28.9179) ccw
  arc A3716 (9.7155, 29.0766) -> (9.7155, 28.7591) centre (9.7155, 28.9179) ccw
  arc A3717 (41.5984, 34.3217) -> (41.5984, 34.0042) centre (41.5984, 34.163) ccw
  arc A3718 (40.1368, 34.3936) -> (39.9123, 34.6182) centre (40.0246, 34.5059) ccw
  arc A3719 (51.5597, 30.2912) -> (51.3352, 30.0667) centre (51.4475, 30.179) ccw
  arc A3720 (52.7108, 27.8914) -> (52.8089, 27.5894) centre (52.7599, 27.7404) ccw
  arc A3721 (54.2254, 27.7608) -> (54.0388, 27.5039) centre (54.1321, 27.6323) ccw
  line L1326 (40.0245, 34.5059) -> (39.1541, 33.6355)
  line L1327 (23.5113, 29.3393) -> (23.0899, 28.9179)
  arc A3722 (39.2664, 33.0383) -> (39.0418, 33.2628) centre (39.1541, 33.1506) ccw
  arc A3723 (27.0833, 31.0152) -> (26.8588, 31.2397) centre (26.9711, 31.1275) ccw
  arc A3724 (47.7497, 34.1012) -> (47.5252, 33.8767) centre (47.6375, 33.9889) ccw
  arc A3725 (25.5874, 30.3851) -> (25.3629, 30.1606) centre (25.4751, 30.2728) ccw
  line L1328 (23.5113, 29.4594) -> (23.5113, 29.3393)
  arc A3726 (37.6266, 31.4642) -> (37.6266, 31.7817) centre (37.6266, 31.623) ccw
  line L1329 (47.2174, 34.163) -> (41.5984, 34.163)
  arc A3727 (41.3677, 34.6181) -> (41.1432, 34.3936) centre (41.2555, 34.5058) ccw
  line L1330 (25.7958, 29.9522) -> (25.4752, 30.2728)
  line L1331 (27.7126, 31.623) -> (27.2925, 31.449)
  arc A3728 (41.2555, 34.3471) -> (41.2555, 34.6646) centre (41.2555, 34.5058) ccw
  arc A3729 (38.9954, 33.1505) -> (39.3128, 33.1505) centre (39.1541, 33.1505) ccw
  arc A3730 (27.2318, 31.5957) -> (27.3533, 31.3023) centre (27.2926, 31.449) ccw
  line L1332 (26.971, 31.1275) -> (26.0225, 30.179)
  arc A3731 (53.4838, 28.0079) -> (53.4341, 27.6943) centre (53.459, 27.8511) ccw
  arc A3732 (39.3128, 33.6355) -> (38.9954, 33.6355) centre (39.1541, 33.6355) ccw
  arc A3733 (40.0245, 34.6646) -> (40.0245, 34.3471) centre (40.0245, 34.5058) ccw
  arc A3734 (51.3352, 30.0667) -> (51.5597, 30.2912) centre (51.4475, 30.179) ccw
  arc A3735 (52.2621, 27.621) -> (52.4488, 27.3641) centre (52.3555, 27.4925) ccw
  arc A3736 (25.6835, 30.0645) -> (25.908, 29.84) centre (25.7958, 29.9522) ccw
  arc A3737 (51.9157, 29.9182) -> (51.6223, 29.7967) centre (51.769, 29.8575) ccw
  line L1333 (51.943, 29.4374) -> (51.769, 29.8575)
  arc A3738 (48.0712, 33.7797) -> (47.8467, 33.5552) centre (47.959, 33.6675) ccw
  line L1334 (23.0899, 28.9179) -> (9.7155, 28.9179)
  line L1335 (39.1541, 33.1505) -> (37.6266, 31.623)
  arc A3739 (23.8488, 29.8594) -> (23.5555, 29.9809) centre (23.7022, 29.9202) ccw
  line L1336 (52.3555, 27.4926) -> (52.2496, 27.3867)
  arc A3740 (54.3805, 27.2121) -> (54.605, 27.4366) centre (54.4928, 27.3244) ccw
  line L1337 (51.4475, 30.179) -> (47.959, 33.6675)
  line L1338 (47.959, 33.6675) -> (47.6375, 33.989)
  line L1339 (26.0225, 30.179) -> (25.7958, 29.9522)
  line L1340 (41.2555, 34.5059) -> (40.0245, 34.5059)
  arc A3741 (23.6236, 29.227) -> (23.399, 29.4515) centre (23.5113, 29.3393) ccw
  arc A3742 (23.0899, 28.7591) -> (23.0899, 29.0766) centre (23.0899, 28.9179) ccw
  line L1341 (54.1321, 27.6324) -> (53.9201, 27.7404)
  arc A3743 (53.34, 25.2413) -> (53.34, 25.5588) centre (53.34, 25.4001) ccw
  arc A3744 (52.0553, 27.8056) -> (51.8307, 27.5811) centre (51.943, 27.6934) ccw
  line L1342 (52.2496, 27.3867) -> (51.943, 27.6933)
  line L1343 (51.943, 27.6933) -> (51.943, 29.4374)
  line L1344 (51.769, 29.8575) -> (51.4475, 30.179)
  arc A3745 (52.1373, 27.499) -> (52.3619, 27.2744) centre (52.2496, 27.3867) ccw
  arc A3746 (52.1373, 27.2744) -> (52.3619, 27.499) centre (52.2496, 27.3867) ccw
  line L1345 (53.4589, 27.8511) -> (53.34, 27.8511)
  arc A3747 (53.34, 27.6923) -> (53.34, 28.0098) centre (53.34, 27.8511) ccw
  line L1346 (53.34, 27.8511) -> (53.2211, 27.8511)
  line L1347 (52.7599, 27.7404) -> (52.5479, 27.6324)
  line L1348 (47.6375, 33.989) -> (47.2174, 34.163)
  arc A3748 (25.4144, 30.1262) -> (25.5359, 30.4195) centre (25.4752, 30.2728) ccw
  line L1349 (70.3249, 35.8521) -> (70.4098, 35.7672)
  arc A3749 (71.9424, 38.0051) -> (71.7179, 37.7806) centre (71.8302, 37.8928) ccw
  arc A3750 (23.5899, 30.0324) -> (23.8144, 29.8079) centre (23.7021, 29.9202) ccw
  line L1350 (25.0144, 30.4637) -> (24.5156, 30.4637)
  line L1351 (41.5984, 34.163) -> (41.2555, 34.5059)
  arc A3751 (27.7734, 31.4763) -> (27.6519, 31.7697) centre (27.7127, 31.623) ccw
  line L1352 (23.7022, 29.9202) -> (23.5113, 29.4594)
  arc A3752 (26.0225, 30.3377) -> (26.0225, 30.0202) centre (26.0225, 30.179) ccw
  arc A3753 (26.1348, 30.0667) -> (25.9103, 30.2912) centre (26.0225, 30.179) ccw
  arc A3754 (41.4861, 34.0507) -> (41.7106, 34.2752) centre (41.5984, 34.1629) ccw
  arc A3755 (27.1298, 31.1275) -> (26.8123, 31.1275) centre (26.9711, 31.1275) ccw
  arc A3756 (24.5764, 30.317) -> (24.4549, 30.6104) centre (24.5157, 30.4637) ccw
  arc A3757 (72.3295, 37.6009) -> (72.0362, 37.4794) centre (72.1829, 37.5401) ccw
  line L1353 (70.8706, 38.0837) -> (70.4098, 37.8928)
  arc A3758 (70.3491, 38.0395) -> (70.4706, 37.7462) centre (70.4099, 37.8929) ccw
  line L1354 (70.4098, 37.8928) -> (70.3249, 37.8079)
  line L1355 (24.5156, 30.4637) -> (24.0548, 30.2728)
  line L1356 (24.0548, 30.2728) -> (23.7022, 29.9202)
  arc A3759 (53.9953, 37.8057) -> (54.1168, 37.5124) centre (54.0561, 37.6591) ccw
  arc A3760 (54.1683, 37.5468) -> (53.9438, 37.7713) centre (54.0561, 37.6591) ccw
  arc A3761 (26.0225, 30.0202) -> (26.0225, 30.3377) centre (26.0225, 30.179) ccw
  arc A3762 (70.8706, 38.2424) -> (70.8706, 37.9249) centre (70.8706, 38.0837) ccw
  arc A3763 (27.7126, 31.7817) -> (27.7126, 31.4642) centre (27.7126, 31.623) ccw
  arc A3764 (25.6835, 29.84) -> (25.908, 30.0645) centre (25.7958, 29.9522) ccw
  arc A3765 (23.3646, 29.5201) -> (23.658, 29.3986) centre (23.5113, 29.4593) ccw
  arc A3766 (47.2174, 34.0042) -> (47.2174, 34.3217) centre (47.2174, 34.163) ccw
  arc A3767 (26.8123, 31.1275) -> (27.1298, 31.1275) centre (26.9711, 31.1275) ccw
  line L1357 (39.1541, 33.6355) -> (39.1541, 33.1505)
  arc A3768 (25.9103, 30.2912) -> (26.1348, 30.0667) centre (26.0225, 30.179) ccw
  arc A3769 (23.6701, 29.4594) -> (23.3526, 29.4594) centre (23.5113, 29.4594) ccw
  arc A3770 (52.1271, 32.4045) -> (52.4446, 32.4045) centre (52.2858, 32.4045) ccw
  arc A3771 (70.9314, 37.937) -> (70.8099, 38.2304) centre (70.8707, 38.0837) ccw
  arc A3772 (72.5204, 36.5199) -> (72.227, 36.6414) centre (72.3737, 36.5806) ccw
  line L1358 (37.6266, 31.623) -> (27.7126, 31.623)
  line L1359 (27.2925, 31.449) -> (26.971, 31.1275)
  line L1360 (25.4752, 30.2728) -> (25.0144, 30.4637)
  arc A3773 (25.0751, 30.6104) -> (24.9536, 30.317) centre (25.0144, 30.4637) ccw
  arc A3774 (70.2126, 37.9202) -> (70.4372, 37.6956) centre (70.3249, 37.8079) ccw
  arc A3775 (72.0362, 36.1806) -> (72.3295, 36.0591) centre (72.1829, 36.1198) ccw
  arc A3776 (72.5324, 37.0794) -> (72.2149, 37.0794) centre (72.3736, 37.0794) ccw
  arc A3777 (72.227, 37.0186) -> (72.5204, 37.1401) centre (72.3737, 37.0793) ccw
  arc A3778 (37.5143, 31.7353) -> (37.7388, 31.5107) centre (37.6266, 31.623) ccw
  arc A3779 (9.5567, 28.9179) -> (9.8742, 28.9179) centre (9.7155, 28.9179) ccw
  line L1361 (54.4155, 37.8079) -> (54.0561, 37.659)
  line L1362 (71.8302, 37.8928) -> (71.3694, 38.0837)
  arc A3780 (27.4048, 31.3367) -> (27.1803, 31.5612) centre (27.2926, 31.449) ccw
  line L1363 (53.781, 37.3839) -> (50.9029, 34.5059)
  arc A3781 (26.8588, 31.2397) -> (27.0833, 31.0152) centre (26.9711, 31.1275) ccw
  line L1364 (9.7155, 28.9179) -> (9.7155, 30.078)
  arc A3782 (54.4155, 37.9666) -> (54.4155, 37.6491) centre (54.4155, 37.8079) ccw
  arc A3783 (24.5156, 30.6224) -> (24.5156, 30.3049) centre (24.5156, 30.4637) ccw
  line L1365 (70.3249, 37.8079) -> (54.4155, 37.8079)
  arc A3784 (23.9941, 30.4195) -> (24.1156, 30.1262) centre (24.0549, 30.2728) ccw
  arc A3785 (39.0418, 33.7477) -> (39.2664, 33.5232) centre (39.1541, 33.6355) ccw
  line L1366 (72.1828, 36.1198) -> (72.3737, 36.5806)
  arc A3786 (70.4706, 35.9138) -> (70.3491, 35.6205) centre (70.4099, 35.7672) ccw
  arc A3787 (72.2149, 36.5806) -> (72.5324, 36.5806) centre (72.3736, 36.5806) ccw
  arc A3788 (24.1671, 30.1606) -> (23.9426, 30.3851) centre (24.0548, 30.2728) ccw
  arc A3789 (23.3526, 29.3393) -> (23.6701, 29.3393) centre (23.5113, 29.3393) ccw
  arc A3790 (25.0144, 30.3049) -> (25.0144, 30.6224) centre (25.0144, 30.4637) ccw
  arc A3791 (54.4762, 37.6612) -> (54.3547, 37.9546) centre (54.4155, 37.8079) ccw
  arc A3792 (72.517, 13.1763) -> (72.517, 13.4938) centre (72.517, 13.335) ccw
  arc A3793 (5.9114, 14.1288) -> (5.9114, 13.8113) centre (5.9114, 13.9701) ccw
  arc A3794 (84.2253, 13.8113) -> (84.2253, 14.1288) centre (84.2253, 13.9701) ccw
  arc A3795 (10.273, 14.1288) -> (10.273, 13.8113) centre (10.273, 13.9701) ccw
  arc A3796 (83.8894, 13.4938) -> (83.8894, 13.1763) centre (83.8894, 13.335) ccw
  arc A3797 (75.452, 11.9063) -> (75.452, 12.2238) centre (75.452, 12.0651) ccw
  arc A3798 (44.4663, 13.8113) -> (44.4663, 14.1288) centre (44.4663, 13.9701) ccw
  arc A3799 (16.7064, 14.7637) -> (16.7064, 14.4463) centre (16.7064, 14.605) ccw
  arc A3800 (72.517, 13.4938) -> (72.517, 13.1763) centre (72.517, 13.335) ccw
  arc A3801 (82.282, 14.1288) -> (82.282, 13.8113) centre (82.282, 13.9701) ccw
  arc A3802 (13.7736, 14.4463) -> (13.7736, 14.7637) centre (13.7736, 14.605) ccw
  arc A3803 (0.7747, 14.7637) -> (0.7747, 14.4463) centre (0.7747, 14.605) ccw
  arc A3804 (14.4467, 12.5413) -> (14.4467, 12.8588) centre (14.4467, 12.7001) ccw
  arc A3805 (84.2253, 13.1763) -> (84.2253, 13.4938) centre (84.2253, 13.335) ccw
  arc A3806 (79.488, 13.4938) -> (79.488, 13.1763) centre (79.488, 13.335) ccw
  arc A3807 (47.512, 14.4463) -> (47.512, 14.7637) centre (47.512, 14.605) ccw
  arc A3808 (70.598, 12.8588) -> (70.598, 12.5413) centre (70.598, 12.7001) ccw
  arc A3809 (73.7489, 12.2238) -> (73.7489, 11.9063) centre (73.7489, 12.0651) ccw
  arc A3810 (71.2851, 11.9063) -> (71.2851, 12.2238) centre (71.2851, 12.0651) ccw
  arc A3811 (21.717, 14.4463) -> (21.717, 14.7637) centre (21.717, 14.605) ccw
  arc A3812 (84.2253, 12.5413) -> (84.2253, 12.8588) centre (84.2253, 12.7001) ccw
  arc A3813 (76.087, 12.5413) -> (76.087, 12.8588) centre (76.087, 12.7001) ccw
  arc A3814 (72.517, 11.9063) -> (72.517, 12.2238) centre (72.517, 12.0651) ccw
  arc A3815 (71.2851, 12.5413) -> (71.2851, 12.8588) centre (71.2851, 12.7001) ccw
  arc A3816 (46.814, 14.7637) -> (46.814, 14.4463) centre (46.814, 14.605) ccw
  arc A3817 (25.7464, 12.8588) -> (25.7464, 12.5413) centre (25.7464, 12.7001) ccw
  arc A3818 (44.7421, 11.9063) -> (44.7421, 12.2238) centre (44.7421, 12.0651) ccw
  arc A3819 (69.328, 14.1288) -> (69.328, 13.8113) centre (69.328, 13.9701) ccw
  arc A3820 (68.693, 14.7637) -> (68.693, 14.4463) centre (68.693, 14.605) ccw
  arc A3821 (46.6979, 12.2238) -> (46.6979, 11.9063) centre (46.6979, 12.0651) ccw
  arc A3822 (0.7747, 14.1288) -> (0.7747, 13.8113) centre (0.7747, 13.9701) ccw
  arc A3823 (8.142, 13.1763) -> (8.142, 13.4938) centre (8.142, 13.335) ccw
  arc A3824 (11.543, 12.8588) -> (11.543, 12.5413) centre (11.543, 12.7001) ccw
  arc A3825 (72.517, 12.5413) -> (72.517, 12.8588) centre (72.517, 12.7001) ccw
  arc A3826 (46.6979, 12.8588) -> (46.6979, 12.5413) centre (46.6979, 12.7001) ccw
  arc A3827 (81.1911, 12.5413) -> (81.1911, 12.8588) centre (81.1911, 12.7001) ccw
  arc A3828 (71.233, 12.2238) -> (71.233, 11.9063) centre (71.233, 12.0651) ccw
  arc A3829 (67.832, 12.5413) -> (67.832, 12.8588) centre (67.832, 12.7001) ccw
  arc A3830 (4.2867, 12.5413) -> (4.2867, 12.8588) centre (4.2867, 12.7001) ccw
  arc A3831 (13.7541, 15.0813) -> (13.7541, 15.3987) centre (13.7541, 15.24) ccw
  arc A3832 (81.1911, 11.9063) -> (81.1911, 12.2238) centre (81.1911, 12.0651) ccw
  arc A3833 (9.003, 15.3987) -> (9.003, 15.0813) centre (9.003, 15.24) ccw
  arc A3834 (21.6335, 15.0813) -> (21.6335, 15.3987) centre (21.6335, 15.24) ccw
  arc A3835 (16.0714, 14.1288) -> (16.0714, 13.8113) centre (16.0714, 13.9701) ccw
  arc A3836 (3.6136, 14.4463) -> (3.6136, 14.7637) centre (3.6136, 14.605) ccw
  arc A3837 (21.2436, 13.8113) -> (21.2436, 14.1288) centre (21.2436, 13.9701) ccw
  arc A3838 (3.5941, 15.0813) -> (3.5941, 15.3987) centre (3.5941, 15.24) ccw
  arc A3839 (77.992, 14.4463) -> (77.992, 14.7637) centre (77.992, 14.605) ccw
  arc A3840 (24.4764, 14.1288) -> (24.4764, 13.8113) centre (24.4764, 13.9701) ccw
  arc A3841 (84.2253, 14.4463) -> (84.2253, 14.7637) centre (84.2253, 14.605) ccw
  arc A3842 (84.2253, 15.7163) -> (84.2253, 16.0338) centre (84.2253, 15.875) ccw
  arc A3843 (3.6136, 15.7163) -> (3.6136, 16.0338) centre (3.6136, 15.875) ccw
  arc A3844 (14.4086, 13.8113) -> (14.4086, 14.1288) centre (14.4086, 13.9701) ccw
  arc A3845 (13.7736, 15.7163) -> (13.7736, 16.0338) centre (13.7736, 15.875) ccw
  arc A3846 (26.7135, 15.0813) -> (26.7135, 15.3987) centre (26.7135, 15.24) ccw
  arc A3847 (49.008, 16.0338) -> (49.008, 15.7163) centre (49.008, 15.875) ccw
  arc A3848 (68.404, 16.0338) -> (68.404, 15.7163) centre (68.404, 15.875) ccw
  arc A3849 (34.2465, 15.3987) -> (34.2465, 15.0813) centre (34.2465, 15.24) ccw
  arc A3850 (46.9737, 14.1288) -> (46.9737, 13.8113) centre (46.9737, 13.9701) ccw
  arc A3851 (24.003, 14.7637) -> (24.003, 14.4463) centre (24.003, 14.605) ccw
  arc A3852 (39.8168, 15.0813) -> (39.8168, 15.3987) centre (39.8168, 15.24) ccw
  arc A3853 (4.2486, 16.3513) -> (4.2486, 16.6688) centre (4.2486, 16.51) ccw
  arc A3854 (0.7747, 16.6688) -> (0.7747, 16.3513) centre (0.7747, 16.51) ccw
  arc A3855 (77.357, 13.8113) -> (77.357, 14.1288) centre (77.357, 13.9701) ccw
  arc A3856 (44.626, 14.4463) -> (44.626, 14.7637) centre (44.626, 14.605) ccw
  arc A3857 (49.643, 15.3987) -> (49.643, 15.0813) centre (49.643, 15.24) ccw
  arc A3858 (83.4507, 15.3987) -> (83.4507, 15.0813) centre (83.4507, 15.24) ccw
  arc A3859 (7.507, 13.8113) -> (7.507, 14.1288) centre (7.507, 13.9701) ccw
  arc A3860 (36.8735, 15.0813) -> (36.8735, 15.3987) centre (36.8735, 15.24) ccw
  arc A3861 (8.368, 16.0338) -> (8.368, 15.7163) centre (8.368, 15.875) ccw
  arc A3862 (83.5279, 16.0338) -> (83.5279, 15.7163) centre (83.5279, 15.875) ccw
  arc A3863 (75.0912, 15.3987) -> (75.0912, 15.0813) centre (75.0912, 15.24) ccw
  arc A3864 (48.147, 13.8113) -> (48.147, 14.1288) centre (48.147, 13.9701) ccw
  arc A3865 (70.1386, 15.7163) -> (70.1386, 16.0338) centre (70.1386, 15.875) ccw
  arc A3866 (73.3702, 13.4938) -> (73.3702, 13.1763) centre (73.3702, 13.335) ccw
  arc A3867 (21.2123, 15.7163) -> (21.2123, 16.0338) centre (21.2123, 15.875) ccw
  arc A3868 (76.722, 13.1763) -> (76.722, 13.4938) centre (76.722, 13.335) ccw
  arc A3869 (82.917, 14.7637) -> (82.917, 14.4463) centre (82.917, 14.605) ccw
  arc A3870 (4.2486, 13.8113) -> (4.2486, 14.1288) centre (4.2486, 13.9701) ccw
  arc A3871 (9.638, 14.7637) -> (9.638, 14.4463) centre (9.638, 14.605) ccw
  arc A3872 (0.7747, 15.3987) -> (0.7747, 15.0813) centre (0.7747, 15.24) ccw
  arc A3873 (81.4646, 13.1763) -> (81.4646, 13.4938) centre (81.4646, 13.335) ccw
  arc A3874 (84.2253, 15.0813) -> (84.2253, 15.3987) centre (84.2253, 15.24) ccw
  arc A3875 (46.877, 15.0813) -> (46.877, 15.3987) centre (46.877, 15.24) ccw
  arc A3876 (40.64, 15.3987) -> (40.64, 15.0813) centre (40.64, 15.24) ccw
  arc A3877 (47.738, 17.3038) -> (47.738, 16.9862) centre (47.738, 17.145) ccw
  arc A3878 (0.7747, 17.9388) -> (0.7747, 17.6212) centre (0.7747, 17.78) ccw
  arc A3879 (31.7935, 17.6212) -> (31.7935, 17.9388) centre (31.7935, 17.78) ccw
  arc A3880 (36.7865, 15.3987) -> (36.7865, 15.0813) centre (36.7865, 15.24) ccw
  arc A3881 (83.5279, 16.6688) -> (83.5279, 16.3513) centre (83.5279, 16.51) ccw
  arc A3882 (40.64, 16.0338) -> (40.64, 15.7163) centre (40.64, 15.875) ccw
  arc A3883 (83.5279, 17.3038) -> (83.5279, 16.9862) centre (83.5279, 17.145) ccw
  arc A3884 (68.5637, 16.6688) -> (68.5637, 16.3513) centre (68.5637, 16.51) ccw
  arc A3885 (0.7747, 16.0338) -> (0.7747, 15.7163) centre (0.7747, 15.875) ccw
  arc A3886 (78.627, 15.0813) -> (78.627, 15.3987) centre (78.627, 15.24) ccw
  arc A3887 (31.7065, 17.9388) -> (31.7065, 17.6212) centre (31.7065, 17.78) ccw
  arc A3888 (34.3335, 15.0813) -> (34.3335, 15.3987) centre (34.3335, 15.24) ccw
  line L1367 (29.1665, 17.78) -> (29.2535, 17.78)
  arc A3889 (5.9114, 16.6688) -> (5.9114, 16.3513) centre (5.9114, 16.51) ccw
  arc A3890 (73.3464, 15.0813) -> (73.3464, 15.3987) centre (73.3464, 15.24) ccw
  arc A3891 (29.2535, 15.0813) -> (29.2535, 15.3987) centre (29.2535, 15.24) ccw
  arc A3892 (40.64, 15.0813) -> (40.64, 15.3987) centre (40.64, 15.24) ccw
  arc A3893 (16.7064, 16.0338) -> (16.7064, 15.7163) centre (16.7064, 15.875) ccw
  arc A3894 (48.373, 16.6688) -> (48.373, 16.3513) centre (48.373, 16.51) ccw
  arc A3895 (53.34, 17.3038) -> (53.34, 16.9862) centre (53.34, 17.145) ccw
  line L1368 (31.7065, 17.78) -> (31.7935, 17.78)
  arc A3896 (29.1665, 15.3987) -> (29.1665, 15.0813) centre (29.1665, 15.24) ccw
  arc A3897 (21.2123, 16.9862) -> (21.2123, 17.3038) centre (21.2123, 17.145) ccw
  arc A3898 (21.0947, 16.3513) -> (21.0947, 16.6688) centre (21.0947, 16.51) ccw
  line L1369 (34.2465, 17.78) -> (34.3335, 17.78)
  arc A3899 (34.3335, 17.6212) -> (34.3335, 17.9388) centre (34.3335, 17.78) ccw
  arc A3900 (46.242, 15.7163) -> (46.242, 16.0338) centre (46.242, 15.875) ccw
  arc A3901 (68.8685, 16.9862) -> (68.8685, 17.3038) centre (68.8685, 17.145) ccw
  arc A3902 (42.0126, 17.3038) -> (42.0126, 16.9862) centre (42.0126, 17.145) ccw
  arc A3903 (21.6335, 17.6212) -> (21.6335, 17.9388) centre (21.6335, 17.78) ccw
  arc A3904 (39.3265, 15.3987) -> (39.3265, 15.0813) centre (39.3265, 15.24) ccw
  arc A3905 (57.037, 16.3513) -> (57.037, 16.6688) centre (57.037, 16.51) ccw
  arc A3906 (26.6265, 17.9388) -> (26.6265, 17.6212) centre (26.6265, 17.78) ccw
  arc A3907 (40.64, 15.7163) -> (40.64, 16.0338) centre (40.64, 15.875) ccw
  line L1370 (26.6265, 17.78) -> (26.7135, 17.78)
  arc A3908 (24.1735, 15.0813) -> (24.1735, 15.3987) centre (24.1735, 15.24) ccw
  arc A3909 (53.34, 16.9862) -> (53.34, 17.3038) centre (53.34, 17.145) ccw
  arc A3910 (41.4632, 15.3987) -> (41.4632, 15.0813) centre (41.4632, 15.24) ccw
  arc A3911 (16.7259, 15.3987) -> (16.7259, 15.0813) centre (16.7259, 15.24) ccw
  arc A3912 (31.7935, 15.0813) -> (31.7935, 15.3987) centre (31.7935, 15.24) ccw
  arc A3913 (26.6265, 15.3987) -> (26.6265, 15.0813) centre (26.6265, 15.24) ccw
  arc A3914 (42.0126, 16.0338) -> (42.0126, 15.7163) centre (42.0126, 15.875) ccw
  arc A3915 (14.4086, 16.3513) -> (14.4086, 16.6688) centre (14.4086, 16.51) ccw
  arc A3916 (24.0865, 15.3987) -> (24.0865, 15.0813) centre (24.0865, 15.24) ccw
  arc A3917 (31.7065, 15.3987) -> (31.7065, 15.0813) centre (31.7065, 15.24) ccw
  arc A3918 (57.672, 15.7163) -> (57.672, 16.0338) centre (57.672, 15.875) ccw
  arc A3919 (51.9547, 16.6688) -> (51.9547, 16.3513) centre (51.9547, 16.51) ccw
  arc A3920 (84.2253, 16.3513) -> (84.2253, 16.6688) centre (84.2253, 16.51) ccw
  line L1371 (24.0865, 17.78) -> (24.1735, 17.78)
  arc A3921 (69.5036, 16.3513) -> (69.5036, 16.6688) centre (69.5036, 16.51) ccw
  arc A3922 (49.6453, 18.8912) -> (49.6453, 19.2088) centre (49.6453, 19.05) ccw
  arc A3923 (52.5445, 18.8912) -> (52.5445, 19.2088) centre (52.5445, 19.05) ccw
  arc A3924 (39.3265, 17.9388) -> (39.3265, 17.6212) centre (39.3265, 17.78) ccw
  arc A3925 (29.1665, 17.9388) -> (29.1665, 17.6212) centre (29.1665, 17.78) ccw
  arc A3926 (54.7705, 18.5738) -> (54.7705, 18.2562) centre (54.7705, 18.415) ccw
  arc A3927 (83.5279, 17.9388) -> (83.5279, 17.6212) centre (83.5279, 17.78) ccw
  arc A3928 (52.5445, 16.3513) -> (52.5445, 16.6688) centre (52.5445, 16.51) ccw